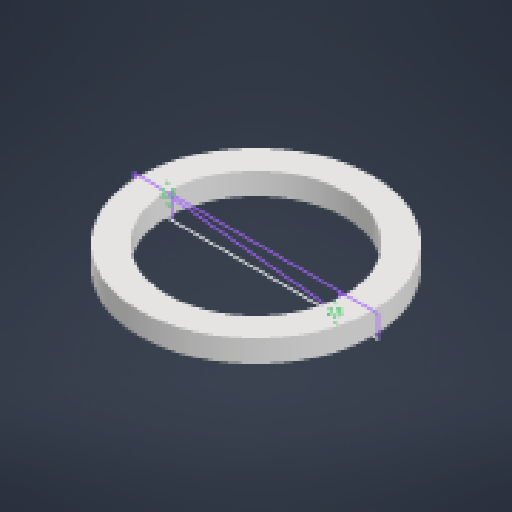
# Autodesk Inventor part: outerspinner
Saved by Autodesk Inventor 2026 (Build 300175050, 175E)
## iProperties
Created: 2026-03-26
Part Number: outerspinner
Material: Generic
Document SubType Name: Modeling
Designer: sniel
Density: 1 g/cm^3
Appearance: Default
Author: sniel
Autodesk Inventor part; units mm, degrees
ref_plane "YZ Plane" through (0, 0, 0) normal (1, 0, 0) x (0, 1, 0)
ref_plane "XZ Plane" through (0, 0, 0) normal (0, 1, 0) x (-1, 0, 0)
ref_plane "XY Plane" through (0, 0, 0) normal (0, 0, 1) x (1, 0, 0)
sketch "Sketch1" plane through (0, 0, 0) normal (0, 1, 0) x (-1, 0, 0)
  circle A0 centre (0, 0) radius 80
  circle A1 centre (0, 0) radius 110
  dimension "d0" = 160
  dimension "d1" = 220
  constraints: 2 centre point, 1 coincident
  measures "d0" diameter of A0
  measures "d1" diameter of A1
extrude "Extrusion1" add sketch "Sketch1" along normal blind 20
sketch "Sketch2" plane through (0, 0, 0) normal (0, 0, 1) x (1, 0, 0)
  line L0 (110, 20) -> (-110, 20)
  line L1 (110, 0) -> (-110, 0)
  line L2 (-75, 20) -> (-75, 0)
  line L3 (75, 20) -> (75, 0)
  line L4 (-110, 0) -> (-110, 20)
  line L5 (110, 0) -> (110, 20)
  line L6 (-75, 20) -> (-75, 17.5)
  line L7 (-75, 17.5) -> (-110, 17.5)
  line L8 (75, 0) -> (75, 2.5)
  line L9 (75, 2.5) -> (-75, 17.5)
  dimension "d6" = 2.5
  dimension "d7" = 2.5
  constraints: 20 end point, 3 point on line, 1 perpendicular
  measures "d6" distance of L2.start L6.end
  measures "d7" distance of L3.end L8.end
body "Solid1"
